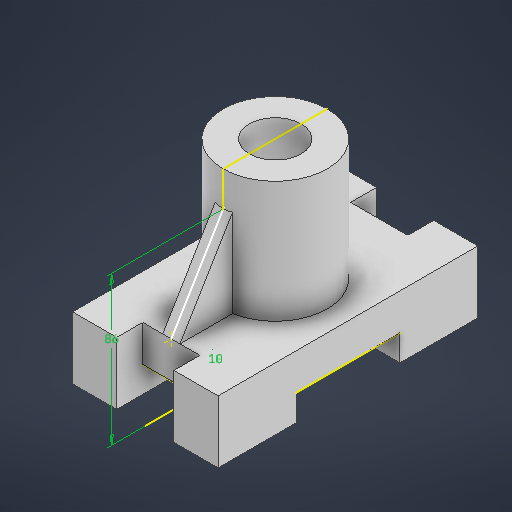
# Autodesk Inventor part: B4
Saved by Autodesk Inventor 2025.4 (Build 294407000, 407)
## iProperties
Created: 2026-05-14
Part Number: B4
Material: Generic
Document SubType Name: Modeling
Designer: VuQuan
Density: 1 g/cm^3
Appearance: Default
Author: VuQuan
Autodesk Inventor part; units mm, degrees
ref_plane "YZ Plane" through (0, 0, 0) normal (1, 0, 0) x (0, 1, 0)
ref_plane "XZ Plane" through (0, 0, 0) normal (0, 1, 0) x (-1, 0, 0)
ref_plane "XY Plane" through (0, 0, 0) normal (0, 0, 1) x (1, 0, 0)
sketch "Sketch1" plane through (0, 0, 0) normal (0, 1, 0) x (-1, 0, 0)
  line L0 (42, -30) -> (42, 75)
  line L1 (42, 75) -> (16.5, 75)
  line L2 (16.5, 75) -> (16.5, 60)
  line L3 (16.5, 60) -> (0, 60)
  line L4 (16.5, 30) -> (42, 30)
  line L5 (0, 0) -> (42, 0) construction
  line L6 (0, 0) -> (0, 60)
  line L7 (-42, -30) -> (-42, 75)
  line L8 (-42, 75) -> (-16.5, 75)
  line L9 (-16.5, 75) -> (-16.5, 60)
  line L10 (-16.5, 60) -> (0, 60)
  line L11 (-16.5, 30) -> (-42, 30)
  line L12 (42, -30) -> (42, -75)
  line L13 (42, -75) -> (16.5, -75)
  line L14 (16.5, -75) -> (16.5, -60)
  line L15 (16.5, -60) -> (0, -60)
  line L16 (-42, -30) -> (-42, -75)
  line L17 (-42, -75) -> (-16.5, -75)
  line L18 (-16.5, -75) -> (-16.5, -60)
  line L19 (-16.5, -60) -> (0, -60)
  line L20 (-42, -30) -> (-16.5, -30)
  line L21 (16.5, -30) -> (42, -30)
  line L22 (16.5, -60) -> (16.5, -30)
  line L23 (-16.5, -60) -> (-16.5, -30)
  line L24 (-16.5, 60) -> (-16.5, 30)
  line L25 (16.5, 60) -> (16.5, 30)
  circle A0 centre (0, 0) radius 15
  line L26 (15, 0) -> (0, -15)
  line L27 (0, -15) -> (-15, 0)
  line L28 (-15, 0) -> (0, 15)
  line L29 (0, 15) -> (15, 0)
  circle A1 centre (0, 0) radius 30
  dimension "d2" = 60
  dimension "d3" = 33
  dimension "d4" = 150
  dimension "d5" = 84
  dimension "d6" = 15
  dimension "d13" = 30
  dimension "d14" = 60
  constraints: 60 end point, 17 symmetric about line, 8 perpendicular, 8 point on line, 4 collinear, 4 point on circle, 2 centre point, 2 coincident, 2 parallel, 2 vertical, 1 horizontal
  measures "d2" diameter of L4 L5
  measures "d3" diameter of L2 L6
  measures "d4" diameter of L1 L5
  measures "d5" diameter of L0 L6
  measures "d6" distance between parallel lines of L3 L1
  measures "d13" diameter of A0
  measures "d14" diameter of A1
extrude "Extrusion1" add sketch "Sketch1" along normal blind 36 contours L12 L13 L14 L22 L21 | L4 L25 L2 L1 L0 | L18 L17 L16 L20 L23 | L24 L11 L7 L8 L9
extrude "Extrusion2" add sketch "Sketch1" against normal blind 21 from surface at 36 contours L21 L22 L15 L19 L23 L20 L7 L11 L24 L10 L3 L25 L4 L0 | L29 A0 | A0 L26 | L28 A0 | A0 L27 | A1
extrude "Extrusion3" add sketch "Sketch1" along normal blind 70 from surface at 36 contours A1
sketch "Sketch4" plane through (-16.5, 15, 60) normal (0, -1, 0) x (1, 0, 0)
  line L0 (1.5, -60) -> (16.5, -45) projected
  line L1 (16.5, -45) -> (31.5, -60) projected
  line L2 (31.5, -60) -> (16.5, -75) projected
  line L3 (16.5, -75) -> (1.5, -60) projected
  line L4 (33, 0) -> (0, 0) projected
  line L5 (0, 0) -> (0, -30) projected
  line L6 (0, -30) -> (-25.5, -30) projected
  line L7 (-25.5, -30) -> (-25.5, -90) projected
  line L8 (-25.5, -90) -> (0, -90) projected
  line L9 (0, -90) -> (0, -120) projected
  line L10 (0, -120) -> (33, -120) projected
  line L11 (33, -120) -> (33, -90) projected
  line L12 (33, -90) -> (58.5, -90) projected
  line L13 (58.5, -90) -> (58.5, -30) projected
  line L14 (58.5, -30) -> (33, -30) projected
  line L15 (33, -30) -> (33, 0) projected
  circle A0 centre (16.5, -25) radius 5
  line L16 (16.5, -60) -> (16.5, 0) projected
  point P0 (16.5, -30)
  dimension "d48" = 10
  constraints: 2 vertical alignment, 1 midpoint, 1 point on line, 2 other
sketch "Sketch2" plane through (0, 0, 0) normal (1, 0, 0) x (0, 1, 0)
  line L0 (36, 30) -> (106, 30) projected
  line L1 (0, 30) -> (15, 30) projected
  line L2 (36, 60) -> (86, 30)
  line L3 (86, 30) -> (106, 18)
  line L4 (0, 75) -> (0, 30) projected
  line L5 (106, 30) -> (106, -30) projected
  point P0 (0, 0)
  dimension "d31" = 86
  constraints: 4 end point, 2 point on line, 1 collinear
  measures "d31" distance from line of L4 L2.end
extrude "Rib1" add sketch "Sketch2" along normal mid plane 10 rib yes fills toward (60.9743, 44.9571) open curves L2 L3
body "Solid1"
